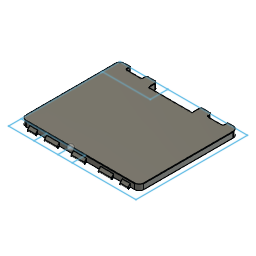
крышка (Autodesk Fusion 360 design; units mm, degrees)
Autodesk Fusion 360 part; units mm, degrees
sketch "Sketch1" plane through (0, 0, 0) normal (0, 1, 0) x (1, 0, 0)
  line L0 (-185, 155) -> (-185, -155)
  line L1 (-185, -155) -> (185, -155)
  line L2 (185, -155) -> (185, 155)
  line L3 (-182.7, -152.7) -> (182.7, -152.7)
  line L4 (182.7, -152.7) -> (182.7, 152.7)
  line L5 (-182.7, 152.7) -> (-182.7, -152.7)
  line L6 (185, 155) -> (153, 155)
  line L7 (153, 155) -> (153, 140)
  line L8 (153, 140) -> (102, 140)
  line L9 (102, 140) -> (102, 141.5866)
  line L10 (102, 141.5866) -> (102, 155)
  line L11 (0, 157.0515) -> (0, 165)
  line L12 (185, 155) -> (153, 155)
  line L13 (182.7, 152.7) -> (153, 152.7)
  line L14 (-153, 155) -> (-153, 140)
  line L15 (-153, 140) -> (-102, 140)
  line L16 (-102, 140) -> (-102, 155)
  line L17 (-153, 155) -> (-185, 155)
  line L18 (-153, 152.7) -> (-182.7, 152.7)
  line L19 (102, 155) -> (69, 155)
  line L20 (69, 155) -> (69, 127)
  line L21 (69, 127) -> (0, 127)
  line L22 (-69, 155) -> (-69, 127)
  line L23 (-69, 127) -> (0, 127)
  line L24 (102, 155) -> (69, 155)
  line L25 (-69, 155) -> (-102, 155)
  line L26 (102, 152.7) -> (69, 152.7)
  line L27 (-69, 152.7) -> (-102, 152.7)
  line L28 (154.5, 155) -> (154.5, 138.5)
  line L29 (154.5, 138.5) -> (100.5, 138.5)
  line L30 (100.5, 138.5) -> (100.5, 141.5866)
  line L31 (100.5, 141.5866) -> (100.5, 155)
  line L32 (-70.5, 155) -> (-70.5, 125.5)
  line L33 (-70.5, 125.5) -> (0, 125.5)
  line L34 (70.5, 125.5) -> (0, 125.5)
  line L35 (70.5, 155) -> (70.5, 125.5)
  line L36 (-154.5, 155) -> (-154.5, 138.5)
  line L37 (-154.5, 138.5) -> (-100.5, 138.5)
  line L38 (-100.5, 138.5) -> (-100.5, 155)
  line L39 (101, 153.5) -> (69, 153.5)
  line L40 (-69, 153.5) -> (-101, 153.5)
  line L41 (-153, 153.5) -> (-183.5, 153.5)
  line L42 (-183.5, 153.5) -> (-183.5, -153.5)
  line L43 (-183.5, -153.5) -> (183.5, -153.5)
  line L44 (183.5, -153.5) -> (183.5, 153.5)
  line L45 (183.5, 153.5) -> (153, 153.5)
  dimension "d1" = 370
  dimension "d2" = 310
  dimension "d11" = 32
  dimension "d12" = 15
  dimension "d13" = 51
  dimension "d15" = 28
  dimension "d17" = -1.5
  dimension "d18" = -1.5
  dimension "d19" = 1.5
  dimension "d20" = -1.5
  dimension "d21" = -1.5
  dimension "d22" = -1.5
  constraint horizontal L12
  constraint perpendicular L0 L17
  constraint parallel L1 L12
  constraint parallel L0 L2
  constraint perpendicular L2 L6
  constraint perpendicular L7 L13
  constraint perpendicular L7 L8
  constraint perpendicular L8 L9
  constraint perpendicular L10 L24
  constraint perpendicular L11 L25
  constraint collinear L12 L24
  constraint coincident L7 L13.end
  constraint coincident L10 L26.start
  constraint collinear L13 L26
  constraint symmetric L6.end L11 L14.start
  constraint symmetric L7.end L11 L14.end
  constraint symmetric L8.end L11 L15.end
  constraint symmetric L10.end L11 L16.end
  constraint collinear L17 L25
  constraint coincident L16 L27.end
  constraint coincident L14 L18.start
  constraint collinear L18 L27
  constraint perpendicular L20 L21
  constraint symmetric L11 L19.end L22.start
  constraint symmetric L11 L20.end L22.end
  constraint symmetric L11 L21.end L23.end
  constraint collinear L24 L25
  constraint coincident L20 L26.end
  constraint coincident L22 L27.start
  constraint collinear L26 L27
  measures "d1" distance of L0.end L1.end
  measures "d2" distance of L0.start L0.end
  measures "d11" distance of L2.end L6.end
  measures "d12" distance of L6.end L7.end
  measures "d13" distance of L7.end L8.end
  measures "d15" distance of L19.end L20.end
extrude "Extrude1" add sketch "Sketch1" along normal blind 3
extrude "Extrude4" add sketch "Sketch1" against normal blind 15 contours L0 L1 L2 L6 L12 L17 L28 L36 L41 L42 L43 L44 L45 | L14 L17 L36 L41 | L14 L18 L36 L41 | L14 L15 L16 L18 L27 L36 L37 L38 | L6 L7 L12 L28 L45 | L7 L13 L28 L45 | L7 L8 L9 L10 L13 L26 L28 L29 L30 L31 | L16 L25 L27 L38 | L22 L27 L32 L40 | L20 L21 L22 L23 L26 L27 L32 L33 L34 L35 | L25 L32 L38 L40 | L22 L25 L32 L40 | L10 L19 L24 L26 L31 | L20 L26 L35 L39 | L19 L24 L31 L35 L39 | L19 L20 L24 L35 L39
sketch "Sketch2" plane through (-185, 0, 0) normal (-1, 0, 0) x (0, 0, 1)
  line L0 (155, -15) -> (155, 3)
  line L1 (155, 3) -> (-155, 3)
  line L2 (-155, 3) -> (-155, -15)
  line L3 (-155, -15) -> (155, -15)
  line L4 (155, -15) -> (158, -15)
  line L5 (158, -15) -> (159.6, -15)
  circle A0 centre (159.6, -15) radius 1.6
  circle A1 centre (159.6, -15) radius 3.4355
  line L6 (155, -4.988) -> (162.1189, -12.6638)
  dimension "d25" = 3
  dimension "d73" = 3.2
  constraint coincident L0.start L3.end
  constraint perpendicular L0 L4
  constraint parallel L4 L5
  constraint coincident L5.end A0.centre
  constraint coincident L4.end A0
  constraint concentric A0 A1
  constraint coincident L0 L6.start
  constraint coincident A1 L6.end
  constraint tangent A1 L6
  measures "d25" distance of L0.start L4.end
  measures "d73" diameter of A0
extrude "Extrude5" add sketch "Sketch2" along normal blind -27 and the other way blind 52 contours L0 L4 A1 L6 | A1
extrude "Extrude6" add sketch "Sketch2" along normal blind -120 and the other way blind 80 contours L0 L4 A1 L6 | A1
extrude "Extrude7" add sketch "Sketch2" along normal blind -164 and the other way blind 205 contours L0 L4 A1 L6 | A1
extrude "Extrude8" add sketch "Sketch2" along normal blind -290 and the other way blind 249 contours L0 L4 A1 L6 | A1
extrude "Extrude9" add sketch "Sketch2" along normal blind -342 and the other way blind 317 contours L0 L4 A1 L6 | A1
fillet "Fillet1" radius 14.5 4 edges at (-183.5, -7.5, 153.5) (-185, -6, 155) (185, -6, 155) (183.5, -7.5, 153.5)
fillet "Fillet2" radius 14.5 4 edges at (185, -6, -155) (183.5, -7.5, -153.5) (-183.5, -7.5, -153.5) (-185, -6, -155)
fillet "Fillet3" radius 5 8 edges at (-102, -6, -155) (-69, -6, -155) (-100.5, -7.5, -153.5) (-70.5, -7.5, -153.5) (100.5, -7.5, -153.5) (70.5, -7.5, -153.5) (69, -6, -155) (102, -6, -155)
sketch "Sketch3" plane through (0, -15, 0) normal (0, -1, 0) x (1, 0, 0)
  line L0 (-154.5, -153.5) -> (-169, -153.5)
  arc A0 (-183.5, -139) -> (-169, -153.5) centre (-169, -139) ccw
  line L1 (-183.5, -139) -> (-183.5, 139)
  arc A1 (-169, 153.5) -> (-183.5, 139) centre (-169, 139) ccw
  line L2 (-169, 153.5) -> (169, 153.5)
  arc A2 (183.5, 139) -> (169, 153.5) centre (169, 139) ccw
  line L3 (183.5, 139) -> (183.5, -139)
  arc A3 (169, -153.5) -> (183.5, -139) centre (169, -139) ccw
  line L4 (169, -153.5) -> (154.5, -153.5)
  line L5 (154.5, -153.5) -> (154.5, -138.5)
  line L6 (154.5, -138.5) -> (100.5, -138.5)
  line L7 (100.5, -138.5) -> (100.5, -148.5)
  arc A4 (95.5, -153.5) -> (100.5, -148.5) centre (95.5, -148.5) ccw
  line L8 (95.5, -153.5) -> (75.5, -153.5)
  arc A5 (70.5, -148.5) -> (75.5, -153.5) centre (75.5, -148.5) ccw
  line L9 (70.5, -148.5) -> (70.5, -125.5)
  line L10 (70.5, -125.5) -> (-70.5, -125.5)
  line L11 (-70.5, -125.5) -> (-70.5, -148.5)
  arc A6 (-75.5, -153.5) -> (-70.5, -148.5) centre (-75.5, -148.5) ccw
  line L12 (-75.5, -153.5) -> (-95.5, -153.5)
  arc A7 (-100.5, -148.5) -> (-95.5, -153.5) centre (-95.5, -148.5) ccw
  line L13 (-100.5, -148.5) -> (-100.5, -138.5)
  line L14 (-100.5, -138.5) -> (-154.5, -138.5)
  line L15 (-154.5, -138.5) -> (-154.5, -153.5)
  arc A8 (97, -155) -> (102, -150) centre (97, -150) ccw
  line L16 (102, -150) -> (102, -140)
  line L17 (102, -140) -> (153, -140)
  line L18 (153, -140) -> (153, -155)
  line L19 (153, -155) -> (170.5, -155)
  arc A9 (170.5, -155) -> (185, -140.5) centre (170.5, -140.5) ccw
  line L20 (185, -140.5) -> (185, 140.5)
  arc A10 (185, 140.5) -> (170.5, 155) centre (170.5, 140.5) ccw
  line L21 (170.5, 155) -> (157, 155)
  line L22 (157, 155) -> (157, 156.1645)
  line L23 (157, 156.1645) -> (132, 156.1645)
  line L24 (132, 156.1645) -> (132, 155)
  line L25 (132, 155) -> (105, 155)
  line L26 (105, 155) -> (105, 156.1645)
  line L27 (105, 156.1645) -> (64, 156.1645)
  line L28 (64, 156.1645) -> (64, 155)
  line L29 (64, 155) -> (20, 155)
  line L30 (20, 155) -> (20, 156.1645)
  line L31 (20, 156.1645) -> (-21, 156.1645)
  line L32 (-21, 156.1645) -> (-21, 155)
  line L33 (-21, 155) -> (-65, 155)
  line L34 (-65, 155) -> (-65, 156.1645)
  line L35 (-65, 156.1645) -> (-105, 156.1645)
  line L36 (-105, 156.1645) -> (-105, 155)
  line L37 (-105, 155) -> (-133, 155)
  line L38 (-133, 155) -> (-133, 156.1645)
  line L39 (-133, 156.1645) -> (-158, 156.1645)
  line L40 (-158, 156.1645) -> (-158, 155)
  line L41 (-158, 155) -> (-170.5, 155)
  arc A11 (-170.5, 155) -> (-185, 140.5) centre (-170.5, 140.5) ccw
  line L42 (-185, 140.5) -> (-185, -140.5)
  arc A12 (-185, -140.5) -> (-170.5, -155) centre (-170.5, -140.5) ccw
  line L43 (-170.5, -155) -> (-153, -155)
  line L44 (-153, -155) -> (-153, -140)
  line L45 (-153, -140) -> (-102, -140)
  line L46 (-102, -140) -> (-102, -150)
  arc A13 (-102, -150) -> (-97, -155) centre (-97, -150) ccw
  line L47 (-97, -155) -> (-74, -155)
  arc A14 (-74, -155) -> (-69, -150) centre (-74, -150) ccw
  line L48 (-69, -150) -> (-69, -127)
  line L49 (-69, -127) -> (69, -127)
  line L50 (69, -127) -> (69, -150)
  arc A15 (69, -150) -> (74, -155) centre (74, -150) ccw
  line L51 (74, -155) -> (97, -155)
  line L52 (0, -140) -> (0, -150)
  line L53 (118, -150) -> (102, -150)
  line L54 (118, -140) -> (118, -150)
  line L55 (102, -140) -> (118, -140)
  line L56 (-118, -148) -> (-102, -148)
  line L57 (118, -148) -> (102, -148)
  line L58 (-102, -140) -> (-102, -148)
  line L59 (-118, -148) -> (-118, -140)
  line L60 (-102, -140) -> (-118, -140)
  line L61 (-118, -146) -> (-102, -146)
  dimension "d63" = -2
  dimension "d65" = 8
  dimension "d66" = 16
  constraint perpendicular L49 L52
  constraint coincident L46 L56.end
  constraint perpendicular L46 L56
  constraint symmetric L52 L56.start L57.start
  constraint symmetric L52 L56.end L57.end
  constraint coincident L45.end L46.start
  constraint coincident L45 L59.end
  constraint perpendicular L45 L59
  measures "d65" distance of L56.start L59.end
  measures "d66" distance of L45.end L59.end
extrude "Extrude10" add sketch "Sketch3" against normal blind 2.5 contours L16 L53 L54 L57 | L16 L17 L54 L55 L57 | L46 L56 L58 L59 L61 | L45 L46 L58 L59 L60 L61
extrude "Extrude11" add sketch "Sketch3" against normal blind 3 contours L16 L53 L54 L57 | L46 L56 L58 L59 L61
sketch "Sketch4" plane through (0, -15, 0) normal (0, -1, 0) x (1, 0, 0)
  line L0 (-200, -115) -> (-50, -115)
  line L1 (-50, -115) -> (-50, -170)
  line L2 (-50, -170) -> (-200, -170)
  line L3 (-200, -170) -> (-200, -115)
  line L4 (-200, -115) -> (-200, -110)
  line L5 (-200, -110) -> (-200, 180)
  line L6 (-200, 180) -> (200, 180)
  line L7 (200, 180) -> (200, -170)
  line L8 (200, -170) -> (-50, -170)
  line L9 (0, 180) -> (0, 140)
  line L10 (0, 140) -> (-200, 140)
  line L11 (-120, 180) -> (-120, 140)
  line L12 (-45, 180) -> (-45, 140)
  constraint horizontal L0
  constraint perpendicular L0 L1
  constraint perpendicular L1 L2
  constraint perpendicular L0 L3
  constraint perpendicular L0 L4
  constraint perpendicular L0 L5
  constraint perpendicular L5 L6
  constraint perpendicular L2 L7
  constraint perpendicular L1 L8
  constraint midpoint L6 L9.start
  constraint perpendicular L6 L9
  constraint coincident L5 L10.end
  constraint perpendicular L5 L10
  constraint coincident L6 L11.start
  constraint coincident L10 L11.end
  constraint perpendicular L10 L11
  constraint coincident L6 L12.start
  constraint perpendicular L6 L12
fillet "Fillet5" radius 4 4 edges at (-153, -6, -140) (-154.5, -7.5, -138.5) (-100.5, -7.5, -138.5) (-102, -4.75, -140)
fillet "Fillet6" radius 4 2 edges at (-69, -6, -127) (-70.5, -7.5, -125.5)
fillet "Fillet7" radius 5 4 edges at (153, -6, -140) (154.5, -7.5, -138.5) (100.5, -7.5, -138.5) (102, -4.75, -140)
